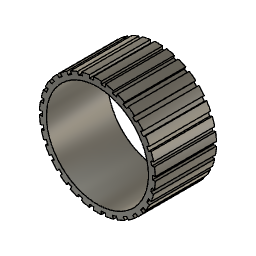
Combined wheel and tire v4 (Autodesk Fusion 360 archive; units mm, degrees)
design "TireFor_Wheels_v1"
Autodesk Fusion 360 part; units mm, degrees
note: some values were not read from the file. Chosen so that the rebuilt part matches the saved one: which face or edge a step refers to; which sketch regions a step uses.
sketch "Sketch1" plane through (0, 0, 0) normal (0, 1, 0) x (1, 0, 0)
  circle A0 centre (0, 0) radius 28.4
  circle A1 centre (0, 0) radius 25
  dimension "d1" = 56.8
  constraint coincident A0.centre A1.centre
  constraint concentric A0 A1
  measures "d1" diameter of A0
extrude "Extrude1" add sketch "Sketch1" against normal blind 30 contours A0 | A1
sketch "Sketch2" plane through (0, 0, 0) normal (1, 0, 0) x (0, 1, 0)
  line L0 (-30, 1, 29) -> (0, 1, 29)
  line L1 (0, 1, 29) -> (0, -1, 29)
  line L2 (0, -1, 29) -> (-30, -1, 29)
  line L3 (-30, -1, 29) -> (-30, 1, 29)
sketch "Sketch2 (curves 29 mm off its plane)" plane through (29, 0, 0) normal (1, 0, 0) x (0, 1, 0)
  line L0 (-30, 1) -> (0, 1)
  line L1 (0, 1) -> (0, -1)
  line L2 (0, -1) -> (-30, -1)
  line L3 (-30, -1) -> (-30, 1)
extrude "Extrude2" cut sketch "Sketch2 (curves 29 mm off its plane)" against normal blind 2
extrude "Extrude3" add sketch "Sketch1" against normal blind 30 contours A1
extrude "Extrude5" cut sketch "Sketch1" against normal blind 46 contours A1
pattern_circular "C-Pattern1" count 30 over 360 about axis through (0, 1.75, 0) along (0, 1, 0) of "Extrude2"
extrude "Extrude4" [suppressed]
